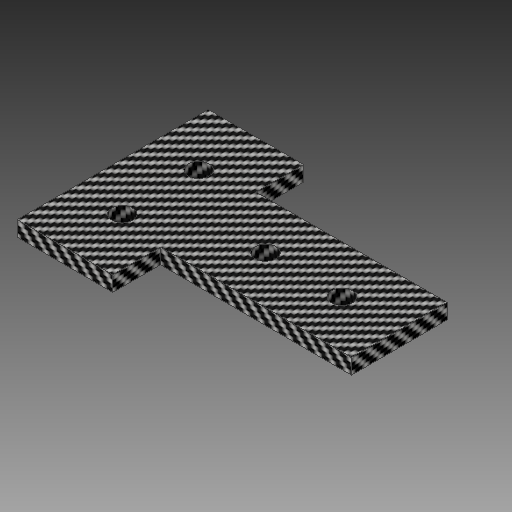
# Autodesk Inventor part: Support Extrusion Brace
Saved by Autodesk Inventor 2019.4 (Build 234330000, 330)
## iProperties
Created: 2019-12-14
Part Number: Support Extrusion Brace
Material: CFRP
Document SubType Name: Modeling
Designer: admin
Density: 1.43 g/cm^3
Appearance: Carbon Fiber
Author: admin
Autodesk Inventor part; units mm, degrees
ref_plane "YZ Plane" through (0, 0, 0) normal (1, 0, 0) x (0, 1, 0)
ref_plane "XZ Plane" through (0, 0, 0) normal (0, 1, 0) x (-1, 0, 0)
ref_plane "XY Plane" through (0, 0, 0) normal (0, 0, 1) x (1, 0, 0)
sketch "Sketch1" plane through (0, 0, 0) normal (0, 1, 0) x (-1, 0, 0)
  line L0 (0, 0) -> (50, 0)
  line L1 (50, 0) -> (50, 12.5)
  line L2 (50, 12.5) -> (75, 12.5)
  line L3 (75, 12.5) -> (75, -37.5)
  line L4 (75, -37.5) -> (50, -37.5)
  line L5 (50, -37.5) -> (50, -25)
  line L6 (50, -25) -> (0, -25)
  line L7 (0, -25) -> (0, 0)
  dimension "d0" = 25
  dimension "d1" = 50
  dimension "d2" = 50
  dimension "d3" = 25
  constraints: 16 end point, 6 perpendicular, 2 point on line, 1 collinear, 1 horizontal
  measures "d0" distance of L6.end L0.start
  measures "d1" distance of L0.start L0.end
  measures "d2" distance of L2.end L3.end
  measures "d3" distance of L1.end L2.end
extrude "Extrusion1" add sketch "Sketch1" along normal blind 4
sketch "Sketch2" plane through (0, 4, 0) normal (0, 1, 0) x (1, 0, 0)
  circle A0 centre (-15, 12.5) radius 2.75 projected
  circle A1 centre (-35, 12.5) radius 2.75 projected
  circle A2 centre (-62.5, 2.5) radius 2.75
  circle A3 centre (-62.5, 22.5) radius 2.75
  line L0 (-75, -12.5) -> (-50, -12.5) projected
  line L1 (-62.5, -12.5) -> (-62.5, 37.5) construction
  line L2 (-50, 37.5) -> (-75, 37.5) projected
  point P0 (0, 0)
  dimension "d6" = 5.5
  dimension "d7" = 5.5
  dimension "d8" = 20
  dimension "d9" = 10
  constraints: 2 centre point, 2 end point, 2 midpoint, 2 point on line
  measures "d6" diameter of A2
  measures "d7" diameter of A3
  measures "d8" distance of A3.centre A2.centre
  measures "d9" vertical distance of A2.centre A1.centre
extrude "Extrusion2" cut sketch "Sketch2" against normal through all
equation "\"d9\" = 0.5 * d8"
body "Solid1"
